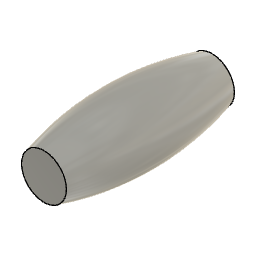
Owl_Body_v3 (Autodesk Fusion 360 design; units mm, degrees)
Autodesk Fusion 360 part; units mm, degrees
note: some values were not read from the file. Set by a fixed rule: which sketch regions a step uses.
sketch "Esquisse1" plane through (0, 0, 0) normal (0, 0, 1) x (1, 0, 0)
  line L0 (0, 0) -> (0, 300)
  line L1 (0, 300) -> (40, 300)
  line L2 (0, 0) -> (40, 0)
  arc A0 (40, 0) -> (40, 300) centre (-479.9533, 150) ccw
  line L3 (0, 0) -> (-59.0933, 0)
  line L4 (-59.0933, 0) -> (-59.0933, 300)
  line L5 (-59.0933, 300) -> (0, 300)
  point P0 (0, 300)
  dimension "d1" = 40
  dimension "d2" = 40
  constraint coincident L0.start L2.start
  constraint coincident P0 L0.end
  constraint vertical L0
  constraint perpendicular L0 L1
  constraint perpendicular L0 L2
  constraint perpendicular L0 L3
  constraint perpendicular L3 L4
  constraint perpendicular L0 L5
  measures "d1" distance of P0 L1.end
  measures "d2" distance of L0.start L2.end
revolve "Révolution1" add sketch "Esquisse1" angle 360 about axis through (0, 0, 0) along (0, 1, 0) contours L0 L1 L2 A0
sketch "Esquisse2" plane through (0, 300, 0) normal (0, 1, 0) x (-1, 0, 0)
  circle A0 centre (0, 0) radius 37.5
  circle A1 centre (0, 0) radius 40
  dimension "d4" = 75
  measures "d4" diameter of A0
extrude "Extrusion1" cut sketch "Esquisse2" against normal blind 290 contours A0
